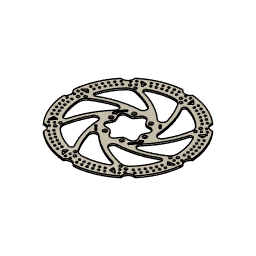
brake disc (Autodesk Fusion 360 design; units mm, degrees)
part number: 2025-07-16-20-32-40-966
Autodesk Fusion 360 part; units mm, degrees
note: some values were not read from the file. Chosen so that the rebuilt part matches the saved one: where a step ends. Set by a fixed rule: which sketch regions a step uses.
sketch "Sketch1" plane through (0, 0, 0) normal (0, 0, 1) x (1, 0, 0)
  circle A0 centre (0, 0) radius 80
  dimension "d1" = 160
  constraint coincident A0.centre origin
  measures "d1" diameter of A0
extrude "Extrude1" add sketch "Sketch1" along normal blind 2
sketch "Sketch2" plane through (0, 0, 2) normal (0, 0, 1) x (-1, 0, 0)
  circle A0 centre (0, 0) radius 80
  circle A1 centre (0, 0) radius 15
  circle A2 centre (0, 0) radius 22.5 construction
  circle A3 centre (0, 0) radius 27.5
  circle A4 centre (22.5, 0) radius 2.5
  circle A5 centre (11.25, 19.4856) radius 2.5
  circle A6 centre (-11.25, 19.4856) radius 2.5
  circle A7 centre (-22.5, 0) radius 2.5
  circle A8 centre (-11.25, -19.4856) radius 2.5
  circle A9 centre (11.25, -19.4856) radius 2.5
  line L0 (23.8157, -13.75) -> (0, 0) construction
  line L1 (0, 0) -> (22.5, 0) construction
  line L2 (23.8157, -13.75) -> (13.3717, 6.7969)
  line L3 (23.8157, -13.75) -> (0.7996, -14.9787)
  line L4 (23.8157, 13.75) -> (13.3717, -6.7969)
  line L5 (23.8157, 13.75) -> (0.7996, 14.9787)
  line L6 (0, 27.5) -> (12.5721, 8.1818)
  line L7 (0, 27.5) -> (-12.5721, 8.1818)
  line L8 (-23.8157, 13.75) -> (-0.7996, 14.9787)
  line L9 (-23.8157, 13.75) -> (-13.3717, -6.7969)
  line L10 (-23.8157, -13.75) -> (-13.3717, 6.7969)
  line L11 (-23.8157, -13.75) -> (-0.7996, -14.9787)
  line L12 (0, -27.5) -> (-12.5721, -8.1818)
  line L13 (0, -27.5) -> (12.5721, -8.1818)
  circle A10 centre (0, 0) radius 64
  line L14 (80, 0) -> (64, 0) construction
  arc A11 (79.7355, 6.5) -> (79.7355, -6.5) centre (83.5229, 0) ccw
  arc A12 (51.7853, 60.9777) -> (60.9777, 51.7853) centre (59.0596, 59.0596) ccw
  arc A13 (-6.5, 79.7355) -> (6.5, 79.7355) centre (0, 83.5229) ccw
  arc A14 (-60.9777, 51.7853) -> (-51.7853, 60.9777) centre (-59.0596, 59.0596) ccw
  arc A15 (-79.7355, -6.5) -> (-79.7355, 6.5) centre (-83.5229, 0) ccw
  arc A16 (-51.7853, -60.9777) -> (-60.9777, -51.7853) centre (-59.0596, -59.0596) ccw
  arc A17 (6.5, -79.7355) -> (-6.5, -79.7355) centre (0, -83.5229) ccw
  arc A18 (60.9777, -51.7853) -> (51.7853, -60.9777) centre (59.0596, -59.0596) ccw
  arc A19 (-21.1814, -17.5385) -> (53.7401, -53.7401) centre (55.8419, 46.2378) ccw
  arc A20 (-17.3302, -14.3497) -> (53.8452, -48.7412) centre (55.8419, 46.2378) ccw
  arc A21 (-2.5759, -27.3791) -> (76, 0) centre (6.7911, 72.1812) ccw
  arc A22 (-2.1076, -22.4011) -> (72.5396, 3.6091) centre (6.7911, 72.1812) ccw
  arc A23 (17.5385, -21.1814) -> (53.7401, 53.7401) centre (-46.2378, 55.8419) ccw
  arc A24 (14.3497, -17.3302) -> (48.7412, 53.8452) centre (-46.2378, 55.8419) ccw
  arc A25 (27.3791, -2.5759) -> (0, 76) centre (-72.1812, 6.7911) ccw
  arc A26 (22.4011, -2.1076) -> (-3.6091, 72.5396) centre (-72.1812, 6.7911) ccw
  arc A27 (21.1814, 17.5385) -> (-53.7401, 53.7401) centre (-55.8419, -46.2378) ccw
  arc A28 (17.3302, 14.3497) -> (-53.8452, 48.7412) centre (-55.8419, -46.2378) ccw
  arc A29 (2.5759, 27.3791) -> (-76, 0) centre (-6.7911, -72.1812) ccw
  arc A30 (2.1076, 22.4011) -> (-72.5396, -3.6091) centre (-6.7911, -72.1812) ccw
  arc A31 (-17.5385, 21.1814) -> (-53.7401, -53.7401) centre (46.2378, -55.8419) ccw
  arc A32 (-14.3497, 17.3302) -> (-48.7412, -53.8452) centre (46.2378, -55.8419) ccw
  arc A33 (-27.3791, 2.5759) -> (0, -76) centre (72.1812, -6.7911) ccw
  arc A34 (-22.4011, 2.1076) -> (3.6091, -72.5396) centre (72.1812, -6.7911) ccw
  circle A35 centre (12.5412, -32.6612) radius 5
  circle A36 centre (31.9629, -14.227) radius 5
  circle A37 centre (32.6612, 12.5412) radius 5
  circle A38 centre (14.227, 31.9629) radius 5
  circle A39 centre (-12.5412, 32.6612) radius 5
  circle A40 centre (-31.9629, 14.227) radius 5
  circle A41 centre (-32.6612, -12.5412) radius 5
  circle A42 centre (-14.227, -31.9629) radius 5
  circle A43 centre (40.0453, -49.9237) radius 1.75
  circle A44 centre (47.0453, -49.9237) radius 1.75
  line L15 (37.2764, -52.0237) -> (25, -52.0237) construction
  line L16 (42.5298, -47.8249) -> (26.5867, -47.8249) construction
  circle A45 centre (50.5453, -54.4237) radius 1.25
  circle A46 centre (43.5453, -54.4237) radius 1.25
  circle A47 centre (47.0453, -58.9237) radius 1.25
  circle A48 centre (35.1725, -66.3425) radius 1.25
  circle A49 centre (32, -62.3425) radius 1.25
  line L17 (43.7764, -61.9237) -> (37.7764, -61.9237)
  line L18 (37.2764, -61.4237) -> (37.2764, -56.9237)
  line L19 (38.0764, -56.5237) -> (44.0764, -61.0237)
  arc A50 (43.7764, -61.9237) -> (44.0764, -61.0237) centre (43.7764, -61.4237) ccw
  arc A51 (38.0764, -56.5237) -> (37.2764, -56.9237) centre (37.7764, -56.9237) ccw
  arc A52 (37.2764, -61.4237) -> (37.7764, -61.9237) centre (37.7764, -61.4237) ccw
  line L20 (0, 0) -> (0, -80) construction
  circle A53 centre (26.8971, -64.708) radius 1.25
  circle A54 centre (29.7386, -68.9496) radius 1.25
  circle A55 centre (21.621, -66.6567) radius 1.25
  circle A56 centre (24.1132, -71.1125) radius 1.25
  circle A57 centre (16.2055, -68.176) radius 1.25
  circle A58 centre (18.3323, -72.8173) radius 1.25
  circle A59 centre (10.6857, -69.2561) radius 1.25
  circle A60 centre (12.4334, -74.053) radius 1.25
  circle A61 centre (5.097, -69.89) radius 1.25
  circle A62 centre (6.4544, -74.8116) radius 1.25
  point P0 (76, 0)
  point P1 (45.2764, -61.9237)
  point P2 (37.2764, -61.9237)
  point P3 (37.2764, -55.9237)
  dimension "d4" = 30
  dimension "d5" = 45
  dimension "d6" = 55
  dimension "d7" = 5
  dimension "d9" = 360
  dimension "d10" = 30
  dimension "d13" = 360
  dimension "d16" = 128
  dimension "d17" = 13
  dimension "d18" = 4
  dimension "d35" = 360
  dimension "d36" = 100
  dimension "d37" = -5
  dimension "d39" = 360
  dimension "d40" = 10
  dimension "d42" = 360
  dimension "d43" = 3.5
  dimension "d44" = 3.5
  dimension "d45" = 4.1988
  dimension "d46" = 2.1
  dimension "d47" = 2.5
  dimension "d48" = 2.5
  dimension "d49" = 2.5
  dimension "d50" = 2.5
  dimension "d51" = 2.5
  dimension "d52" = 8
  dimension "d53" = 6
  dimension "d54" = 0.5
  dimension "d55" = 0.5
  dimension "d56" = 0.5
  dimension "d57" = 4
  dimension "d58" = 7
  dimension "d59" = 4.5
  dimension "d60" = 3.5
  dimension "d61" = 7
  dimension "d62" = 32
  dimension "d63" = 14
  dimension "d64" = 14
  dimension "d65" = 9
  dimension "d66" = 3
  dimension "d68" = -23
  constraint coincident A0.centre A1.centre
  constraint concentric A0 A2
  constraint concentric A1 A3
  constraint coincident A2 A4.centre
  constraint coincident A3 L0.start
  constraint coincident A4.centre L1.end
  constraint horizontal L1
  constraint coincident A1 L2.end
  constraint coincident A1 L3.end
  constraint tangent A1 L3
  constraint tangent A1 L2
  constraint concentric A3 A10
  constraint coincident A0 L14.start
  constraint coincident A10 L14.end
  constraint horizontal L14
  constraint coincident A0 A11.start
  constraint coincident A0 A11.end
  constraint midpoint A11 P0
  constraint horizontal L14.start P0
  constraint coincident A3 A19.start
  constraint midpoint A18 A19.end
  constraint tangent A3 A19
  constraint tangent A20 A35
  constraint tangent A21 A35
  constraint coincident A10 A43.centre
  constraint coincident A19 L15.start
  constraint coincident A10 L15.start
  constraint horizontal L15
  constraint coincident A20 L16.start
  constraint coincident A10 L16.start
  constraint horizontal L16
  constraint horizontal L17
  constraint perpendicular L17 L18
  constraint coincident P1 L17
  constraint coincident P1 L19
  constraint tangent L17 A50
  constraint tangent L19 A50
  constraint coincident P3 L19
  constraint coincident P3 L18
  constraint tangent L19 A51
  constraint tangent L18 A51
  constraint coincident P2 L17
  constraint coincident P2 L18
  constraint tangent L17 A52
  constraint tangent L18 A52
  constraint coincident A0 L20.end
  constraint vertical L20
  constraint horizontal A45.centre A46.centre
  constraint vertical A44.centre A47.centre
  constraint horizontal A43.centre A44.centre
  constraint vertical L15.start L18.end
  measures "d4" diameter of A1
  measures "d5" diameter of A2
  measures "d6" diameter of A3
  measures "d7" diameter of A4
  measures "d10" angle of L0 L1
  measures "d16" diameter of A10
  measures "d17" vertical distance of A11.end A11.start
  measures "d18" distance of L14.start P0
  measures "d36" radius of A19
  measures "d40" diameter of A35
  measures "d43" diameter of A43
  measures "d44" diameter of A44
  measures "d45" distance of L15 L16
  measures "d46" distance of A43.centre L15
  measures "d47" diameter of A45
  measures "d48" diameter of A46
  measures "d49" diameter of A47
  measures "d50" diameter of A48
  measures "d51" diameter of A49
  measures "d52" distance of P1 P2
  measures "d53" distance of P2 P3
  measures "d54" radius of A50
  measures "d55" radius of A51
  measures "d56" radius of A52
  measures "d57" vertical distance of A48.centre A49.centre
  measures "d58" distance of A43.centre A44.centre
  measures "d59" vertical distance of A46.centre A47.centre
  measures "d60" horizontal distance of A45.centre A47.centre
  measures "d61" distance of A45.centre A46.centre
  measures "d62" distance of A49.centre L20
  measures "d63" distance of A46.centre A49.centre
  measures "d64" distance of A47.centre A48.centre
  measures "d65" distance of A44.centre A47.centre
  measures "d66" distance of A47.centre L17
extrude "Extrude3" cut sketch "Sketch2" along normal up to far side of body 1 contours A0 A18 | A19 A45 | A19 A45 | A10 A43 | A10 A43 | A10 A19 A34 A42 | A42 | A20 A44 | A20 A44 | A46 | A47 | A48 | A49 | L17 L18 L19 A50 A51 A52 | A53 | A54 | A55 | A56 | A57 | A58 | A59 | A60 | A61 | A62
pattern_circular "C-Pattern1" count 8 over 360 about axis through (0, 0, 2) along (0, 0, 1) of "Extrude3"
extrude "Extrude4" cut sketch "Sketch2" against normal blind 15 contours A1 L3 L11 L12 L13 | L2 L3 A24 | A1 L11 L12 | A1 L9 L10 L11 L12 A34 | A1 L2 L3 L4 L13 A24 | A1 L3 L13 | L10 L11 A34 | A1 | A1 L2 L4 | A1 L2 L4 L5 L6 A26 | A1 L9 L10 | L4 L5 A26 | A1 L7 L8 L9 L10 A32 | L8 L9 A32 | A1 L5 L6 | A1 L5 L6 L7 L8 | A1 L7 L8 | A4 | A5 A28 | A5 A28 | A6 | A7 | A8 A20 | A8 A20 | A9
fillet "Fillet1" radius 5 1 edges at (8.4133, -14.5722, 1)
fillet "Fillet2" radius 5 5 edges at (-8.4133, -14.5722, 1) (-16.8266, 0, 1) (-8.4133, 14.5722, 1) (16.8266, 0, 1) (8.4133, 14.5722, 1)
fillet "Fillet3" radius 5 6 edges at (-23.8157, -13.75, 1) (0, -27.5, 1) (23.8157, -13.75, 1) (23.8157, 13.75, 1) (0, 27.5, 1) (-23.8157, 13.75, 1)
fillet "Fillet5" radius 3 1 edges at (63.1447, -10.4279, 1)
fillet "Fillet6" radius 10 1 edges at (42.5298, -47.8249, 1)
fillet "Fillet7" radius 1 2 edges at (79.7355, 6.5, 1) (79.7355, -6.5, 1)
pattern_circular "C-Pattern2" count 8 over 360 about axis through (0, 0, 2) along (0, 0, -1) of "Fillet5", "Fillet6", "Fillet7"
sketch "Sketch3" plane through (0, 0, 2) normal (0, 0, 1) x (-1, 0, 0)
  arc A0 (-46.9276, -37.2622) -> (-43.995, -46.4806) centre (-37.1207, -39.218) ccw
  arc A1 (-37.0445, -10.1356) -> (-46.9276, -37.2622) centre (46.2378, -55.8419) ccw
  arc A2 (-27.6687, -12.2674) -> (-37.0445, -10.1356) centre (-32.6612, -12.5412) ccw
  arc A3 (-27.6687, -12.2674) -> (-14.2275, -57.1252) centre (72.1812, -6.7911) ccw
  arc A4 (-17.647, -61.519) -> (-14.2275, -57.1252) centre (-16.8198, -58.6353) ccw
  arc A5 (-43.995, -46.4806) -> (-17.647, -61.519) centre (0, 0) ccw
  arc A6 (37.2622, -46.9276) -> (46.4806, -43.995) centre (39.218, -37.1207) ccw
  arc A7 (10.1356, -37.0445) -> (37.2622, -46.9276) centre (55.8419, 46.2378) ccw
  arc A8 (12.2674, -27.6687) -> (10.1356, -37.0445) centre (12.5412, -32.6612) ccw
  arc A9 (12.2674, -27.6687) -> (57.1252, -14.2275) centre (6.7911, 72.1812) ccw
  arc A10 (61.519, -17.647) -> (57.1252, -14.2275) centre (58.6353, -16.8198) ccw
  arc A11 (46.4806, -43.995) -> (61.519, -17.647) centre (0, 0) ccw
  arc A12 (46.9276, 37.2622) -> (43.995, 46.4806) centre (37.1207, 39.218) ccw
  arc A13 (37.0445, 10.1356) -> (46.9276, 37.2622) centre (-46.2378, 55.8419) ccw
  arc A14 (27.6687, 12.2674) -> (37.0445, 10.1356) centre (32.6612, 12.5412) ccw
  arc A15 (27.6687, 12.2674) -> (14.2275, 57.1252) centre (-72.1812, 6.7911) ccw
  arc A16 (17.647, 61.519) -> (14.2275, 57.1252) centre (16.8198, 58.6353) ccw
  arc A17 (43.995, 46.4806) -> (17.647, 61.519) centre (0, 0) ccw
  circle A18 centre (-40.0453, 49.9237) radius 1.75
  circle A19 centre (-47.0453, 49.9237) radius 1.75
  arc A20 (-7.027, -16.7024) -> (-10.9512, -14.4367) centre (-11.2177, -19.4296) ccw
  line L0 (-10.9512, -14.4367) -> (-16.1437, -14.1596)
  arc A21 (-20.3344, -6.901) -> (-16.1437, -14.1596) centre (-15.8771, -9.1667) ccw
  line L1 (-20.3344, -6.901) -> (-17.9782, -2.2656)
  arc A22 (-17.9782, -2.2656) -> (-17.9782, 2.2656) centre (-22.4354, 0) ccw
  line L2 (-17.9782, 2.2656) -> (-20.3344, 6.901)
  arc A23 (-16.1437, 14.1596) -> (-20.3344, 6.901) centre (-15.8771, 9.1667) ccw
  line L3 (-16.1437, 14.1596) -> (-10.9512, 14.4367)
  arc A24 (-10.9512, 14.4367) -> (-7.027, 16.7024) centre (-11.2177, 19.4296) ccw
  line L4 (-7.027, 16.7024) -> (-4.1907, 21.0606)
  arc A25 (4.1907, 21.0606) -> (-4.1907, 21.0606) centre (0, 18.3333) ccw
  line L5 (4.1907, 21.0606) -> (7.027, 16.7024)
  arc A26 (7.027, 16.7024) -> (10.9512, 14.4367) centre (11.2177, 19.4296) ccw
  line L6 (10.9512, 14.4367) -> (16.1437, 14.1596)
  arc A27 (20.3344, 6.901) -> (16.1437, 14.1596) centre (15.8771, 9.1667) ccw
  line L7 (20.3344, 6.901) -> (17.9782, 2.2656)
  arc A28 (17.9782, 2.2656) -> (17.9782, -2.2656) centre (22.4354, 0) ccw
  line L8 (17.9782, -2.2656) -> (20.3344, -6.901)
  arc A29 (16.1437, -14.1596) -> (20.3344, -6.901) centre (15.8771, -9.1667) ccw
  line L9 (16.1437, -14.1596) -> (10.9512, -14.4367)
  arc A30 (10.9512, -14.4367) -> (7.027, -16.7024) centre (11.2177, -19.4296) ccw
  line L10 (7.027, -16.7024) -> (4.1907, -21.0606)
  arc A31 (-4.1907, -21.0606) -> (4.1907, -21.0606) centre (0, -18.3333) ccw
  line L11 (-4.1907, -21.0606) -> (-7.027, -16.7024)
  circle A32 centre (-11.25, -19.4856) radius 2.5
  circle A33 centre (11.25, -19.4856) radius 2.5
  circle A34 centre (-22.5, 0) radius 2.5
  circle A35 centre (11.25, 19.4856) radius 2.5
  circle A36 centre (22.5, 0) radius 2.5
  circle A37 centre (-11.25, 19.4856) radius 2.5
  circle A38 centre (-2.7425, -74.2243) radius 1.25
  circle A39 centre (-8.3993, -74.9314) radius 1.25
  circle A40 centre (-27.7263, -69.7831) radius 1.25
  circle A41 centre (-38.5267, -64.4525) radius 1.25
  circle A42 centre (-48.3358, -57.4637) radius 1.25
  circle A43 centre (-43.5716, -61.1551) radius 1.25
  circle A44 centre (-31.8451, -62.4218) radius 1.25
  circle A45 centre (-21.4554, -66.7102) radius 1.25
  circle A46 centre (-7.6922, -69.2745) radius 1.25
  circle A47 centre (-2.0354, -68.5674) radius 1.75
  arc A48 (-12.8321, -74.7413) -> (-11.9835, -74.317) centre (-12.4785, -74.3877) ccw
  line L12 (-12.8321, -74.7413) -> (-17.0747, -70.4987)
  arc A49 (-17.0747, -69.7915) -> (-17.0747, -70.4987) centre (-16.7211, -70.1451) ccw
  line L13 (-17.0747, -69.7915) -> (-13.8927, -66.6096)
  arc A50 (-13.0442, -66.8924) -> (-13.8927, -66.6096) centre (-13.5392, -66.9631) ccw
  line L14 (-13.0442, -66.8924) -> (-11.9835, -74.317)
  circle A51 centre (-26.7364, -64.7746) radius 1.25
  circle A52 centre (-36.7487, -59.6668) radius 1.25
  circle A53 centre (-45.8155, -53.0238) radius 1.25
  circle A54 centre (-41.4155, -56.5274) radius 1.25
  circle A55 centre (-33.2336, -67.3347) radius 1.25
  circle A56 centre (-22.0405, -71.782) radius 1.25
  circle A57 centre (-6.9851, -63.6177) radius 1.75
  circle A58 centre (-54.4237, -50.5453) radius 1.25
  circle A59 centre (-58.9237, -47.0453) radius 1.25
  circle A60 centre (-68.9496, -29.7386) radius 1.25
  circle A61 centre (-72.8173, -18.3323) radius 1.25
  circle A62 centre (-74.8116, -6.4544) radius 1.25
  circle A63 centre (-74.053, -12.4334) radius 1.25
  circle A64 centre (-66.6567, -21.621) radius 1.25
  circle A65 centre (-62.3425, -32) radius 1.25
  circle A66 centre (-54.4237, -43.5453) radius 1.25
  circle A67 centre (-49.9237, -47.0453) radius 1.75
  arc A68 (-61.9237, -43.7764) -> (-61.0237, -44.0764) centre (-61.4237, -43.7764) ccw
  line L15 (-61.9237, -43.7764) -> (-61.9237, -37.7764)
  arc A69 (-61.4237, -37.2764) -> (-61.9237, -37.7764) centre (-61.4237, -37.7764) ccw
  line L16 (-61.4237, -37.2764) -> (-56.9237, -37.2764)
  arc A70 (-56.5237, -38.0764) -> (-56.9237, -37.2764) centre (-56.9237, -37.7764) ccw
  line L17 (-56.5237, -38.0764) -> (-61.0237, -44.0764)
  circle A71 centre (-64.708, -26.8971) radius 1.25
  circle A72 centre (-68.176, -16.2055) radius 1.25
  circle A73 centre (-69.89, -5.097) radius 1.25
  circle A74 centre (-69.2561, -10.6857) radius 1.25
  circle A75 centre (-71.1125, -24.1132) radius 1.25
  circle A76 centre (-66.3425, -35.1725) radius 1.25
  circle A77 centre (-49.9237, -40.0453) radius 1.75
  circle A78 centre (-63.6177, 6.9851) radius 1.75
  circle A79 centre (-74.2243, 2.7425) radius 1.25
  circle A80 centre (-74.9314, 8.3993) radius 1.25
  circle A81 centre (-69.7831, 27.7263) radius 1.25
  circle A82 centre (-64.4525, 38.5267) radius 1.25
  circle A83 centre (-57.4637, 48.3358) radius 1.25
  circle A84 centre (-61.1551, 43.5716) radius 1.25
  circle A85 centre (-62.4218, 31.8451) radius 1.25
  circle A86 centre (-66.7102, 21.4554) radius 1.25
  circle A87 centre (-69.2745, 7.6922) radius 1.25
  circle A88 centre (-68.5674, 2.0354) radius 1.75
  arc A89 (-74.7413, 12.8321) -> (-74.317, 11.9835) centre (-74.3877, 12.4785) ccw
  line L18 (-74.7413, 12.8321) -> (-70.4987, 17.0747)
  arc A90 (-69.7915, 17.0747) -> (-70.4987, 17.0747) centre (-70.1451, 16.7211) ccw
  line L19 (-69.7915, 17.0747) -> (-66.6096, 13.8927)
  arc A91 (-66.8924, 13.0442) -> (-66.6096, 13.8927) centre (-66.9631, 13.5392) ccw
  line L20 (-66.8924, 13.0442) -> (-74.317, 11.9835)
  circle A92 centre (-64.7746, 26.7364) radius 1.25
  circle A93 centre (-59.6668, 36.7487) radius 1.25
  circle A94 centre (-53.0238, 45.8155) radius 1.25
  circle A95 centre (-56.5274, 41.4155) radius 1.25
  circle A96 centre (-67.3347, 33.2336) radius 1.25
  circle A97 centre (-71.782, 22.0405) radius 1.25
  circle A98 centre (-50.5453, 54.4237) radius 1.25
  circle A99 centre (-47.0453, 58.9237) radius 1.25
  circle A100 centre (-29.7386, 68.9496) radius 1.25
  circle A101 centre (-18.3323, 72.8173) radius 1.25
  circle A102 centre (-6.4544, 74.8116) radius 1.25
  circle A103 centre (-12.4334, 74.053) radius 1.25
  circle A104 centre (-21.621, 66.6567) radius 1.25
  circle A105 centre (-32, 62.3425) radius 1.25
  circle A106 centre (-43.5453, 54.4237) radius 1.25
  arc A107 (-43.7764, 61.9237) -> (-44.0764, 61.0237) centre (-43.7764, 61.4237) ccw
  line L21 (-43.7764, 61.9237) -> (-37.7764, 61.9237)
  arc A108 (-37.2764, 61.4237) -> (-37.7764, 61.9237) centre (-37.7764, 61.4237) ccw
  line L22 (-37.2764, 61.4237) -> (-37.2764, 56.9237)
  arc A109 (-38.0764, 56.5237) -> (-37.2764, 56.9237) centre (-37.7764, 56.9237) ccw
  line L23 (-38.0764, 56.5237) -> (-44.0764, 61.0237)
  circle A110 centre (-26.8971, 64.708) radius 1.25
  circle A111 centre (-16.2055, 68.176) radius 1.25
  circle A112 centre (-5.097, 69.89) radius 1.25
  circle A113 centre (-10.6857, 69.2561) radius 1.25
  circle A114 centre (-24.1132, 71.1125) radius 1.25
  circle A115 centre (-35.1725, 66.3425) radius 1.25
  circle A116 centre (2.7425, 74.2243) radius 1.25
  circle A117 centre (8.3993, 74.9314) radius 1.25
  circle A118 centre (27.7263, 69.7831) radius 1.25
  circle A119 centre (38.5267, 64.4525) radius 1.25
  circle A120 centre (48.3358, 57.4637) radius 1.25
  circle A121 centre (43.5716, 61.1551) radius 1.25
  circle A122 centre (31.8451, 62.4218) radius 1.25
  circle A123 centre (21.4554, 66.7102) radius 1.25
  circle A124 centre (7.6922, 69.2745) radius 1.25
  circle A125 centre (2.0354, 68.5674) radius 1.75
  arc A126 (12.8321, 74.7413) -> (11.9835, 74.317) centre (12.4785, 74.3877) ccw
  line L24 (12.8321, 74.7413) -> (17.0747, 70.4987)
  arc A127 (17.0747, 69.7915) -> (17.0747, 70.4987) centre (16.7211, 70.1451) ccw
  line L25 (17.0747, 69.7915) -> (13.8927, 66.6096)
  arc A128 (13.0442, 66.8924) -> (13.8927, 66.6096) centre (13.5392, 66.9631) ccw
  line L26 (13.0442, 66.8924) -> (11.9835, 74.317)
  circle A129 centre (26.7364, 64.7746) radius 1.25
  circle A130 centre (36.7487, 59.6668) radius 1.25
  circle A131 centre (45.8155, 53.0238) radius 1.25
  circle A132 centre (41.4155, 56.5274) radius 1.25
  circle A133 centre (33.2336, 67.3347) radius 1.25
  circle A134 centre (22.0405, 71.782) radius 1.25
  circle A135 centre (6.9851, 63.6177) radius 1.75
  circle A136 centre (54.4237, 50.5453) radius 1.25
  circle A137 centre (58.9237, 47.0453) radius 1.25
  circle A138 centre (68.9496, 29.7386) radius 1.25
  circle A139 centre (72.8173, 18.3323) radius 1.25
  circle A140 centre (74.8116, 6.4544) radius 1.25
  circle A141 centre (74.053, 12.4334) radius 1.25
  circle A142 centre (66.6567, 21.621) radius 1.25
  circle A143 centre (62.3425, 32) radius 1.25
  circle A144 centre (54.4237, 43.5453) radius 1.25
  circle A145 centre (49.9237, 47.0453) radius 1.75
  arc A146 (61.9237, 43.7764) -> (61.0237, 44.0764) centre (61.4237, 43.7764) ccw
  line L27 (61.9237, 43.7764) -> (61.9237, 37.7764)
  arc A147 (61.4237, 37.2764) -> (61.9237, 37.7764) centre (61.4237, 37.7764) ccw
  line L28 (61.4237, 37.2764) -> (56.9237, 37.2764)
  arc A148 (56.5237, 38.0764) -> (56.9237, 37.2764) centre (56.9237, 37.7764) ccw
  line L29 (56.5237, 38.0764) -> (61.0237, 44.0764)
  circle A149 centre (64.708, 26.8971) radius 1.25
  circle A150 centre (68.176, 16.2055) radius 1.25
  circle A151 centre (69.89, 5.097) radius 1.25
  circle A152 centre (69.2561, 10.6857) radius 1.25
  circle A153 centre (71.1125, 24.1132) radius 1.25
  circle A154 centre (66.3425, 35.1725) radius 1.25
  circle A155 centre (49.9237, 40.0453) radius 1.75
  circle A156 centre (74.2243, -2.7425) radius 1.25
  circle A157 centre (74.9314, -8.3993) radius 1.25
  circle A158 centre (69.7831, -27.7263) radius 1.25
  circle A159 centre (64.4525, -38.5267) radius 1.25
  circle A160 centre (57.4637, -48.3358) radius 1.25
  circle A161 centre (61.1551, -43.5716) radius 1.25
  circle A162 centre (62.4218, -31.8451) radius 1.25
  circle A163 centre (66.7102, -21.4554) radius 1.25
  circle A164 centre (69.2745, -7.6922) radius 1.25
  circle A165 centre (68.5674, -2.0354) radius 1.75
  arc A166 (74.7413, -12.8321) -> (74.317, -11.9835) centre (74.3877, -12.4785) ccw
  line L30 (74.7413, -12.8321) -> (70.4987, -17.0747)
  arc A167 (69.7915, -17.0747) -> (70.4987, -17.0747) centre (70.1451, -16.7211) ccw
  line L31 (69.7915, -17.0747) -> (66.6096, -13.8927)
  arc A168 (66.8924, -13.0442) -> (66.6096, -13.8927) centre (66.9631, -13.5392) ccw
  line L32 (66.8924, -13.0442) -> (74.317, -11.9835)
  circle A169 centre (64.7746, -26.7364) radius 1.25
  circle A170 centre (59.6668, -36.7487) radius 1.25
  circle A171 centre (53.0238, -45.8155) radius 1.25
  circle A172 centre (56.5274, -41.4155) radius 1.25
  circle A173 centre (67.3347, -33.2336) radius 1.25
  circle A174 centre (71.782, -22.0405) radius 1.25
  circle A175 centre (63.6177, -6.9851) radius 1.75
  circle A176 centre (50.5453, -54.4237) radius 1.25
  circle A177 centre (47.0453, -58.9237) radius 1.25
  circle A178 centre (29.7386, -68.9496) radius 1.25
  circle A179 centre (18.3323, -72.8173) radius 1.25
  circle A180 centre (6.4544, -74.8116) radius 1.25
  circle A181 centre (12.4334, -74.053) radius 1.25
  circle A182 centre (21.621, -66.6567) radius 1.25
  circle A183 centre (32, -62.3425) radius 1.25
  circle A184 centre (43.5453, -54.4237) radius 1.25
  circle A185 centre (47.0453, -49.9237) radius 1.75
  arc A186 (43.7764, -61.9237) -> (44.0764, -61.0237) centre (43.7764, -61.4237) ccw
  line L33 (43.7764, -61.9237) -> (37.7764, -61.9237)
  arc A187 (37.2764, -61.4237) -> (37.7764, -61.9237) centre (37.7764, -61.4237) ccw
  line L34 (37.2764, -61.4237) -> (37.2764, -56.9237)
  arc A188 (38.0764, -56.5237) -> (37.2764, -56.9237) centre (37.7764, -56.9237) ccw
  line L35 (38.0764, -56.5237) -> (44.0764, -61.0237)
  circle A189 centre (26.8971, -64.708) radius 1.25
  circle A190 centre (16.2055, -68.176) radius 1.25
  circle A191 centre (5.097, -69.89) radius 1.25
  circle A192 centre (10.6857, -69.2561) radius 1.25
  circle A193 centre (24.1132, -71.1125) radius 1.25
  circle A194 centre (35.1725, -66.3425) radius 1.25
  circle A195 centre (40.0453, -49.9237) radius 1.75
  arc A196 (-10.1356, 37.0445) -> (-37.2622, 46.9276) centre (-55.8419, -46.2378) ccw
  arc A197 (-12.2674, 27.6687) -> (-10.1356, 37.0445) centre (-12.5412, 32.6612) ccw
  arc A198 (-12.2674, 27.6687) -> (-57.1252, 14.2275) centre (-6.7911, -72.1812) ccw
  arc A199 (-61.519, 17.647) -> (-57.1252, 14.2275) centre (-58.6353, 16.8198) ccw
  arc A200 (-46.4806, 43.995) -> (-61.519, 17.647) centre (0, 0) ccw
  arc A201 (-37.2622, 46.9276) -> (-46.4806, 43.995) centre (-39.218, 37.1207) ccw
  arc A202 (6.8345, 59.5312) -> (-1.7576, 63.9759) centre (-1.483, 53.9796) ccw
  arc A203 (19.0274, 33.3614) -> (6.8345, 59.5312) centre (-72.1812, 6.7911) ccw
  arc A204 (10.8904, 28.2391) -> (19.0274, 33.3614) centre (14.227, 31.9629) ccw
  arc A205 (10.8904, 28.2391) -> (-30.3333, 50.454) centre (-55.8419, -46.2378) ccw
  arc A206 (-31.0222, 55.9788) -> (-30.3333, 50.454) centre (-29.568, 53.3548) ccw
  arc A207 (-1.7576, 63.9759) -> (-31.0222, 55.9788) centre (0, 0) ccw
  arc A208 (59.5312, -6.8345) -> (63.9759, 1.7576) centre (53.9796, 1.483) ccw
  arc A209 (33.3614, -19.0274) -> (59.5312, -6.8345) centre (6.7911, 72.1812) ccw
  arc A210 (28.2391, -10.8904) -> (33.3614, -19.0274) centre (31.9629, -14.227) ccw
  arc A211 (28.2391, -10.8904) -> (50.454, 30.3333) centre (-46.2378, 55.8419) ccw
  arc A212 (55.9788, 31.0222) -> (50.454, 30.3333) centre (53.3548, 29.568) ccw
  arc A213 (63.9759, 1.7576) -> (55.9788, 31.0222) centre (0, 0) ccw
  arc A214 (-6.8345, -59.5312) -> (1.7576, -63.9759) centre (1.483, -53.9796) ccw
  arc A215 (-19.0274, -33.3614) -> (-6.8345, -59.5312) centre (72.1812, -6.7911) ccw
  arc A216 (-10.8904, -28.2391) -> (-19.0274, -33.3614) centre (-14.227, -31.9629) ccw
  arc A217 (-10.8904, -28.2391) -> (30.3333, -50.454) centre (55.8419, 46.2378) ccw
  arc A218 (31.0222, -55.9788) -> (30.3333, -50.454) centre (29.568, -53.3548) ccw
  arc A219 (1.7576, -63.9759) -> (31.0222, -55.9788) centre (0, 0) ccw
  arc A220 (-59.5312, 6.8345) -> (-63.9759, -1.7576) centre (-53.9796, -1.483) ccw
  arc A221 (-33.3614, 19.0274) -> (-59.5312, 6.8345) centre (-6.7911, -72.1812) ccw
  arc A222 (-28.2391, 10.8904) -> (-33.3614, 19.0274) centre (-31.9629, 14.227) ccw
  arc A223 (-28.2391, 10.8904) -> (-50.454, -30.3333) centre (46.2378, -55.8419) ccw
  arc A224 (-55.9788, -31.0222) -> (-50.454, -30.3333) centre (-53.3548, -29.568) ccw
  arc A225 (-63.9759, -1.7576) -> (-55.9788, -31.0222) centre (0, 0) ccw
  arc A226 (-51.6611, -60.4223) -> (-51.3192, -61.3705) centre (-50.6777, -60.6034) ccw
  arc A227 (-51.3192, -61.3705) -> (-7.1074, -79.6837) centre (0, 0) ccw
  arc A228 (-7.1074, -79.6837) -> (-6.1951, -79.2549) centre (-7.0186, -78.6876) ccw
  arc A229 (6.1951, -79.2549) -> (-6.1951, -79.2549) centre (0, -83.5229) ccw
  arc A230 (6.1951, -79.2549) -> (7.1074, -79.6837) centre (7.0186, -78.6876) ccw
  arc A231 (7.1074, -79.6837) -> (51.3192, -61.3705) centre (0, 0) ccw
  arc A232 (51.3192, -61.3705) -> (51.6611, -60.4223) centre (50.6777, -60.6034) ccw
  arc A233 (60.4223, -51.6611) -> (51.6611, -60.4223) centre (59.0596, -59.0596) ccw
  arc A234 (60.4223, -51.6611) -> (61.3705, -51.3192) centre (60.6034, -50.6777) ccw
  arc A235 (61.3705, -51.3192) -> (79.6837, -7.1074) centre (0, 0) ccw
  arc A236 (79.6837, -7.1074) -> (79.2549, -6.1951) centre (78.6876, -7.0186) ccw
  arc A237 (79.2549, 6.1951) -> (79.2549, -6.1951) centre (83.5229, 0) ccw
  arc A238 (79.2549, 6.1951) -> (79.6837, 7.1074) centre (78.6876, 7.0186) ccw
  arc A239 (79.6837, 7.1074) -> (61.3705, 51.3192) centre (0, 0) ccw
  arc A240 (61.3705, 51.3192) -> (60.4223, 51.6611) centre (60.6034, 50.6777) ccw
  arc A241 (51.6611, 60.4223) -> (60.4223, 51.6611) centre (59.0596, 59.0596) ccw
  arc A242 (51.6611, 60.4223) -> (51.3192, 61.3705) centre (50.6777, 60.6034) ccw
  arc A243 (51.3192, 61.3705) -> (7.1074, 79.6837) centre (0, 0) ccw
  arc A244 (7.1074, 79.6837) -> (6.1951, 79.2549) centre (7.0186, 78.6876) ccw
  arc A245 (-6.1951, 79.2549) -> (6.1951, 79.2549) centre (0, 83.5229) ccw
  arc A246 (-6.1951, 79.2549) -> (-7.1074, 79.6837) centre (-7.0186, 78.6876) ccw
  arc A247 (-7.1074, 79.6837) -> (-51.3192, 61.3705) centre (0, 0) ccw
  arc A248 (-51.3192, 61.3705) -> (-51.6611, 60.4223) centre (-50.6777, 60.6034) ccw
  arc A249 (-60.4223, 51.6611) -> (-51.6611, 60.4223) centre (-59.0596, 59.0596) ccw
  arc A250 (-60.4223, 51.6611) -> (-61.3705, 51.3192) centre (-60.6034, 50.6777) ccw
  arc A251 (-61.3705, 51.3192) -> (-79.6837, 7.1074) centre (0, 0) ccw
  arc A252 (-79.6837, 7.1074) -> (-79.2549, 6.1951) centre (-78.6876, 7.0186) ccw
  arc A253 (-79.2549, -6.1951) -> (-79.2549, 6.1951) centre (-83.5229, 0) ccw
  arc A254 (-79.2549, -6.1951) -> (-79.6837, -7.1074) centre (-78.6876, -7.0186) ccw
  arc A255 (-79.6837, -7.1074) -> (-61.3705, -51.3192) centre (0, 0) ccw
  arc A256 (-61.3705, -51.3192) -> (-60.4223, -51.6611) centre (-60.6034, -50.6777) ccw
  arc A257 (-51.6611, -60.4223) -> (-60.4223, -51.6611) centre (-59.0596, -59.0596) ccw
  circle A258 centre (0, 0) radius 26
  circle A259 centre (0, 0) radius 27 construction
  circle A260 centre (0, 0) radius 28
  line L36 (-33.4427, 33.4427) -> (32.6254, -32.6254)
  line L37 (-41.0288, 14.9333) -> (41.3939, -15.0661)
  line L38 (0, 0) -> (-17.4354, 0)
  line L39 (-28.1908, 10.2606) -> (-26.4598, 5.3739)
  line L40 (-26.4598, 5.3739) -> (-22.5526, 8.2085)
  line L41 (28.1908, -10.2606) -> (26.4598, -5.3739)
  line L42 (26.4598, -5.3739) -> (22.5526, -8.2085)
  line L43 (18.1852, 24.611) -> (23.842, 18.9541) construction
  line L44 (23.842, 18.9541) -> (23.8424, 18.9545) construction
  line L45 (23.8424, 18.9545) -> (18.1855, 24.6113) construction
  line L46 (18.1855, 24.6113) -> (18.1852, 24.611) construction
  line L47 (-17.1616, -23.2158) -> (-22.7178, -17.6597) construction
  line L48 (-22.7178, -17.6597) -> (-25.2711, -20.2129) construction
  line L49 (-25.2711, -20.2129) -> (-19.7149, -25.7691) construction
  line L50 (-19.7149, -25.7691) -> (-17.1616, -23.2158) construction
  point P0 (-25.3717, 9.2345)
  dimension "d91" = 52
  dimension "d92" = 54
  dimension "d93" = 56
  dimension "d94" = 45
  dimension "d95" = 25
  dimension "d96" = 4
  dimension "d97" = 6
  dimension "d98" = 3
  dimension "d100" = 360
  dimension "d101" = 2
  dimension "d102" = 2
  text T0 "BRAKE" font "Arial" height 2 align centre middle in box 8 x 0.0005 at (18.1852, 24.611) x (0.707107, -0.707107) y (0.707107, 0.707107) spacing 1.01
  text T1 "DISK" font "Arial" height 2 align centre middle in box 7.8576 x 3.6109 at (-17.1616, -23.2158) x (-0.707107, 0.707107) y (-0.707107, -0.707107) spacing 1.01
  constraint concentric A5 A258
  constraint coincident A5.centre A11.centre
  constraint concentric A5 A260
  constraint coincident A5.centre L36
  constraint coincident A5.centre L37
  constraint midpoint A22 L38.end
  constraint coincident L37 L39.start
  constraint coincident A259 L39.end
  constraint coincident L37 L40.end
  constraint coincident L37 P0
  constraint coincident A259 P0
  measures "d91" diameter of A258
  measures "d92" diameter of A259
  measures "d93" diameter of A260
  measures "d94" angle of L36 L38
  measures "d95" angle of L36 L37
  measures "d96" distance of L37 L39.end
  measures "d97" distance of L39.start L40.end
  measures "d98" distance of L39.start P0
extrude "Extrude5" cut sketch "Sketch3" sketch "Sketch3" against normal blind 0.2 contours A258 A260 L36 L37 | A258 A260 L37 L39 L40 | A258 L37 L40 | A258 L37 L42 | A258 A260 L37 L41 L42 | A258 A260 L36 L37 | A260 L37 L41 | A260 L37 L39 of sketch 2 text T0 T1
extrude "Extrude2" [suppressed]
